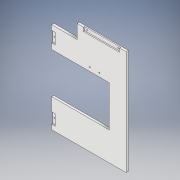
# Autodesk Inventor part: TC001b
Saved by Autodesk Inventor 2017 SP1 (Build 210196100, 196)
## iProperties
Created: 2018-01-07
Part Number: TC001b
Material: ABS Plastic
Document SubType Name: Modeling
Designer: Zach
Density: 1.06 g/cm^3
Appearance: CR White
Author: Zach
Autodesk Inventor part; units mm, degrees
ref_plane "YZ Plane" through (0, 0, 0) normal (1, 0, 0) x (0, 1, 0)
ref_plane "XZ Plane" through (0, 0, 0) normal (0, 1, 0) x (-1, 0, 0)
ref_plane "XY Plane" through (0, 0, 0) normal (0, 0, 1) x (1, 0, 0)
sketch "Sketch1" plane through (0, 0, 0) normal (0, 0, 1) x (1, 0, 0)
  line L0 (0, 0) -> (620, 0)
  line L1 (620, 0) -> (620, 620)
  line L2 (620, 620) -> (0, 620)
  line L3 (0, 620) -> (0, 0)
  line L4 (203.5, 491) -> (416.5, 491)
  line L5 (416.5, 491) -> (416.5, 378)
  line L6 (416.5, 378) -> (203.5, 378)
  line L7 (203.5, 378) -> (203.5, 491)
  line L8 (620, 0) -> (310, 0)
  line L9 (310, 0) -> (310, 435)
  line L10 (310, 435) -> (620, 435)
  line L11 (620, 435) -> (620, 0)
  point P0 (310, 491)
  point P1 (310, 620)
  dimension "d0" = 620
  dimension "d1" = 620
  dimension "d2" = 213
  dimension "d3" = 113
  dimension "d4" = 129
  dimension "d28" = 435
  constraints: 24 end point, 6 parallel, 3 horizontal, 3 perpendicular, 2 midpoint, 2 vertical alignment
  measures "d0" distance of L2.end L1.end
  measures "d1" distance of L1.end L0.end
  measures "d2" distance of L5.end L6.end
  measures "d3" distance of L4.end L5.end
  measures "d4" distance between parallel lines of L2 L4
  measures "d28" distance of L8.end L9.end
extrude "Extrusion1" add sketch "Sketch1" along normal blind 10 contours L3 L2 L1 L10 L5 L4 L7 L6 L9 L0 | L9 L6 L5 L10 L1 L0
sketch "Sketch6" plane through (0, 0, 10) normal (0, 0, 1) x (1, 0, 0)
  line L0 (0, 0) -> (620, 0) projected
  line L1 (620, 0) -> (310, 0)
  line L2 (310, 0) -> (310, 435)
  line L3 (310, 435) -> (620, 435)
  line L4 (620, 435) -> (620, 0)
  line L5 (620, 620) -> (0, 620) projected
  line L6 (620, 435) -> (0, 435)
  line L7 (0, 435) -> (0, 620)
  line L8 (0, 620) -> (620, 620)
  line L9 (620, 620) -> (620, 435)
  line L10 (310, 435) -> (0, 435)
  line L11 (0, 435) -> (0, 0)
  line L12 (0, 0) -> (310, 0)
  line L13 (310, 0) -> (310, 435)
  point P0 (310, 620)
  dimension "d29" = 435
  constraints: 24 end point, 6 parallel, 3 horizontal, 3 perpendicular, 1 midpoint, 1 vertical alignment
  measures "d29" distance of L1.end L2.end
extrude "Extrusion6" cut sketch "Sketch6" against normal through all contours L11 L6 L2 L0 | L7 L5 L9 L3 L6
sketch "Sketch7" plane through (0, 0, 10) normal (0, 0, 1) x (1, 0, 0)
  line L0 (310, 378) -> (310, 0) projected
  line L1 (416.5, 435) -> (620, 435) projected
  line L2 (443.25, 435) -> (593.25, 435)
  line L3 (593.25, 435) -> (593.25, 420)
  line L4 (593.25, 420) -> (443.25, 420)
  line L5 (443.25, 420) -> (443.25, 435)
  line L6 (310, 358) -> (325, 358)
  line L7 (325, 358) -> (325, 313)
  line L8 (325, 313) -> (310, 313)
  line L9 (310, 313) -> (310, 358)
  line L10 (310, 20) -> (325, 20)
  line L11 (325, 20) -> (325, 65)
  line L12 (325, 65) -> (310, 65)
  line L13 (310, 65) -> (310, 20)
  line L14 (416.5, 378) -> (310, 378) projected
  line L15 (310, 0) -> (620, 0) projected
  point P0 (0, 0)
  point P1 (518.25, 435)
  dimension "d34" = 150
  dimension "d35" = 15
  dimension "d48" = 15
  dimension "d49" = 45
  dimension "d50" = 15
  dimension "d51" = 45
  dimension "d52" = 20
  dimension "d53" = 20
  constraints: 24 end point, 6 parallel, 3 horizontal, 3 perpendicular, 3 point on line, 2 midpoint
  measures "d34" distance of L3.end L4.end
  measures "d35" distance of L2.end L3.end
  measures "d48" distance of L7.end L8.end
  measures "d49" distance of L6.end L7.end
  measures "d50" distance of L12.end L11.end
  measures "d51" distance of L11.end L10.end
  measures "d52" distance between parallel lines of L6 L14
  measures "d53" distance between parallel lines of L15 L10
extrude "Extrusion7" cut sketch "Sketch7" against normal blind 5
sketch "Sketch8" plane through (0, 0, 5) normal (0, 0, 1) x (1, 0, 0)
  circle A0 centre (453.25, 427.5) radius 2.5
  circle A1 centre (583.25, 427.5) radius 2.5
  circle A2 centre (317.5, 335.5) radius 2.5
  circle A3 centre (317.5, 42.5) radius 2.5
  line L0 (310, 313) -> (310, 358) projected
  line L1 (325, 313) -> (310, 313) projected
  line L2 (325, 358) -> (325, 313) projected
  line L3 (310, 358) -> (325, 358) projected
  line L4 (443.25, 420) -> (443.25, 435) projected
  line L5 (593.25, 420) -> (443.25, 420) projected
  line L6 (593.25, 435) -> (593.25, 420) projected
  line L7 (443.25, 435) -> (593.25, 435) projected
  line L8 (310, 20) -> (310, 65) projected
  line L9 (325, 20) -> (310, 20) projected
  line L10 (325, 65) -> (325, 20) projected
  line L11 (310, 65) -> (325, 65) projected
  line L12 (310, 20) -> (310, 65) projected
  point P0 (0, 0)
  point P1 (593.25, 427.5)
  point P2 (443.25, 427.5)
  point P3 (317.5, 358)
  point P4 (317.5, 65)
  point P5 (310, 42.5)
  point P6 (310, 335.5)
  dimension "d38" = 5
  dimension "d39" = 5
  dimension "d40" = 5
  dimension "d54" = 10
  dimension "d55" = 10
  constraints: 6 midpoint, 4 centre point, 4 horizontal alignment, 2 vertical alignment
  measures "d38" diameter of A0
  measures "d39" diameter of A1
  measures "d40" diameter of A2
  measures "d54" distance from line of L4 A0.centre
  measures "d55" distance from line of L6 A1.centre
extrude "Extrusion8" cut sketch "Sketch8" against normal through all contours A0 | A1 | A2 | A3
sketch "Sketch9" plane through (0, 0, 10) normal (0, 0, 1) x (1, 0, 0)
  line L0 (550, 289) -> (310, 289)
  line L1 (310, 289) -> (310, 119)
  line L2 (310, 119) -> (550, 119)
  line L3 (550, 119) -> (550, 289)
  line L4 (310, 313) -> (310, 65) projected
  line L5 (325, 313) -> (310, 313) projected
  point P0 (0, 0)
  dimension "d56" = 240
  dimension "d57" = 170
  dimension "d67" = 24
  constraints: 8 end point, 2 parallel, 1 horizontal, 1 perpendicular, 1 point on line
  measures "d56" distance of L2.end L1.end
  measures "d57" distance of L1.end L0.end
  measures "d67" distance between parallel lines of L5 L0
extrude "Extrusion9" cut sketch "Sketch9" against normal through all
sketch "Sketch10" plane through (0, 0, 10) normal (0, 0, 1) x (1, 0, 0)
  circle A0 centre (509, 304) radius 2.5
  circle A1 centre (469, 304) radius 2.5
  line L0 (550, 289) -> (550, 119) projected
  line L1 (310, 289) -> (550, 289) projected
  point P0 (0, 0)
  dimension "d60" = 5
  dimension "d61" = 5
  dimension "d62" = 41
  dimension "d63" = 40
  dimension "d64" = 15
  constraints: 2 centre point, 1 horizontal alignment
  measures "d60" diameter of A0
  measures "d61" diameter of A1
  measures "d62" distance from line of A0.centre L0
  measures "d63" distance of A0.centre A1.centre
  measures "d64" distance from line of L1 A0.centre
extrude "Extrusion10" cut sketch "Sketch10" along normal through all both and the other way through all
chamfer "Chamfer1" distance 10 angle 5 1 edges at (430, 119, 0) measured on face at (430, 119, 0.5)
body "Solid1"
